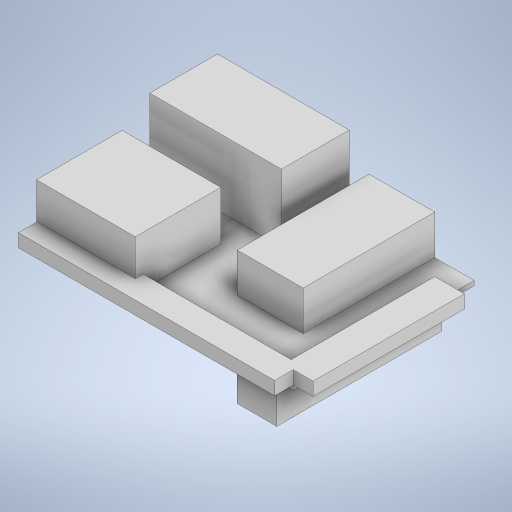
# Autodesk Inventor part: board
Saved by Autodesk Inventor 2023 (Build 270158000, 158)
## iProperties
Created: 2022-04-19
Part Number: board
Material: Generic
Document SubType Name: Modeling
Designer: cooki
Density: 1 g/cm^3
Appearance: Default
Author: cooki
Autodesk Inventor part; units mm, degrees
ref_plane "YZ Plane" through (0, 0, 0) normal (1, 0, 0) x (0, 1, 0)
ref_plane "XZ Plane" through (0, 0, 0) normal (0, 1, 0) x (-1, 0, 0)
ref_plane "XY Plane" through (0, 0, 0) normal (0, 0, 1) x (1, 0, 0)
sketch "Sketch1" plane through (0, 0, 0) normal (0, 1, 0) x (-1, 0, 0)
  line L0 (49.53, 34.925) -> (-49.53, 34.925)
  line L1 (-49.53, 34.925) -> (-49.53, -34.925)
  line L2 (-49.53, -34.925) -> (49.53, -34.925)
  line L3 (49.53, -34.925) -> (49.53, 34.925)
  point P0 (0, 0)
  point P1 (0, -34.925)
  point P2 (49.53, 0)
  dimension "d0" = 99.06
  dimension "d1" = 69.85
  constraints: 8 end point, 2 midpoint, 2 parallel, 1 horizontal, 1 horizontal alignment, 1 perpendicular, 1 vertical alignment
  measures "d0" distance of L2.end L1.end
  measures "d1" distance of L1.end L0.end
extrude "Extrusion1" add sketch "Sketch1" along normal blind 1.778
sketch "Sketch2" plane through (0, 1.778, 0) normal (0, 1, 0) x (1, 0, 0)
  line L0 (-49.53, 34.925) -> (-49.53, -34.925) projected
  line L1 (-49.53, 34.925) -> (1.27, 34.925)
  line L2 (1.27, 34.925) -> (1.27, 8.763)
  line L3 (1.27, 8.763) -> (-49.53, 8.763)
  line L4 (-49.53, 8.763) -> (-49.53, 34.925)
  point P0 (0, 0)
  dimension "d4" = 50.8
  dimension "d5" = 26.162
  constraints: 8 end point, 2 parallel, 1 horizontal, 1 perpendicular
  measures "d4" distance of L2.end L3.end
  measures "d5" distance of L1.end L2.end
extrude "Extrusion2" add sketch "Sketch2" along normal blind 26.162
sketch "Sketch3" plane through (0, 1.778, 0) normal (0, 1, 0) x (1, 0, 0)
  line L0 (-49.53, 34.925) -> (-49.53, -34.925) projected
  line L1 (-49.53, -34.925) -> (-11.43, -34.925)
  line L2 (-11.43, -34.925) -> (-11.43, -1.905)
  line L3 (-11.43, -1.905) -> (-49.53, -1.905)
  line L4 (-49.53, -1.905) -> (-49.53, -34.925)
  point P0 (0, 0)
  dimension "d8" = 38.1
  dimension "d9" = 33.02
  constraints: 8 end point, 2 parallel, 1 horizontal, 1 perpendicular
  measures "d8" distance of L3.end L2.end
  measures "d9" distance of L2.end L1.end
extrude "Extrusion3" add sketch "Sketch3" along normal blind 19.05
sketch "Sketch4" plane through (0, 1.778, 0) normal (0, 1, 0) x (1, 0, 0)
  line L0 (1.27, 34.925) -> (1.27, 8.763) projected
  line L1 (1.27, 34.925) -> (8.89, 34.925)
  line L2 (49.53, 34.925) -> (-49.53, 34.925) projected
  line L3 (8.89, 34.925) -> (34.29, 34.925)
  line L4 (34.29, 34.925) -> (34.29, -15.875)
  line L5 (34.29, -15.875) -> (8.89, -15.875)
  line L6 (8.89, -15.875) -> (8.89, 34.925)
  point P0 (0, 0)
  dimension "d12" = 7.62
  dimension "d13" = 25.4
  dimension "d14" = 50.8
  constraints: 10 end point, 2 parallel, 1 horizontal, 1 perpendicular, 1 point on line
  measures "d12" distance of L0.start L1.end
  measures "d13" distance of L4.end L5.end
  measures "d14" distance of L3.end L4.end
extrude "Extrusion4" add sketch "Sketch4" along normal blind 15.24
sketch "Sketch5" plane through (0, 0, 0) normal (0, -1, 0) x (1, 0, 0)
  line L0 (-11.43, 34.925) -> (49.53, 34.925) projected
  line L1 (49.53, 34.925) -> (43.18, 34.925)
  line L2 (43.18, 34.925) -> (27.94, 34.925)
  line L3 (27.94, 34.925) -> (27.94, -28.575)
  line L4 (27.94, -28.575) -> (43.18, -28.575)
  line L5 (43.18, -28.575) -> (43.18, 34.925)
  point P0 (0, 0)
  dimension "d17" = 6.35
  dimension "d18" = 15.24
  dimension "d19" = 63.5
  constraints: 10 end point, 2 parallel, 1 horizontal, 1 perpendicular, 1 point on line
  measures "d17" distance of L0.end L1.end
  measures "d18" distance of L4.end L3.end
  measures "d19" distance of L3.end L2.end
extrude "Extrusion5" add sketch "Sketch5" along normal blind 15.24
sketch "Sketch6" plane through (0, 1.778, 0) normal (0, 1, 0) x (1, 0, 0)
  line L0 (49.53, -34.925) -> (45.7244, -34.925)
  line L1 (45.7244, -34.925) -> (57.1544, -34.925)
  line L2 (57.1544, -34.925) -> (57.1544, 23.495)
  line L3 (57.1544, 23.495) -> (45.7244, 23.495)
  line L4 (45.7244, 23.495) -> (45.7244, -34.925)
  point P0 (0, 0)
  dimension "d22" = 11.43
  dimension "d23" = 58.42
  constraints: 10 end point, 2 horizontal, 2 parallel, 1 perpendicular
  measures "d22" distance of L3.end L2.end
  measures "d23" distance of L2.end L1.end
extrude "Extrusion6" add sketch "Sketch6" along normal blind 5.08
sketch "Sketch7" plane through (0, 1.778, 0) normal (0, 1, 0) x (1, 0, 0)
  line L0 (49.53, -34.925) -> (49.53, 34.925) projected
  line L1 (49.53, -31.9382) -> (-49.3242, -31.9382)
  line L2 (-49.3242, -31.9382) -> (-49.3242, -42.0982)
  line L3 (-49.3242, -42.0982) -> (49.53, -42.0982)
  line L4 (49.53, -42.0982) -> (49.53, -31.9382)
  point P0 (0, 0)
  dimension "d26" = 10.16
  constraints: 8 end point, 2 parallel, 1 horizontal, 1 perpendicular, 1 point on line
  measures "d26" distance of L2.end L1.end
extrude "Extrusion7" add sketch "Sketch7" along normal blind 5.08
body "Solid1"
